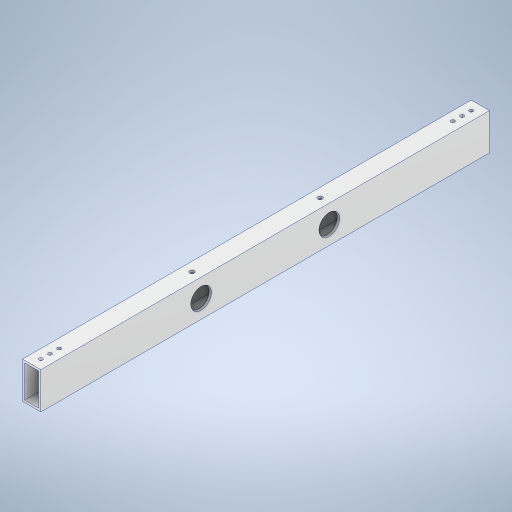
# Autodesk Inventor part: middle_alum_swerve
Saved by Autodesk Inventor 2024 (Build 280153000, 153)
## iProperties
Created: 2023-10-09
Part Number: middle_alum_swerve
Material: Aluminum 6061
Document SubType Name: Modeling
Designer: s137416
Density: 2.7 g/cm^3
Appearance: Aluminum - Flat
Author: s137416
Autodesk Inventor part; units mm, degrees
ref_plane "YZ Plane" through (0, 0, 0) normal (1, 0, 0) x (0, 1, 0)
ref_plane "XZ Plane" through (0, 0, 0) normal (0, 1, 0) x (-1, 0, 0)
ref_plane "XY Plane" through (0, 0, 0) normal (0, 0, 1) x (1, 0, 0)
sketch "Sketch1" plane through (0, 0, 0) normal (0, 1, 0) x (-1, 0, 0)
  line L0 (5.8164, 600.598) -> (-19.5836, 600.598)
  line L1 (-19.5836, 600.598) -> (-19.5836, -21.702)
  line L2 (-19.5836, -21.702) -> (5.8164, -21.702)
  line L3 (5.8164, -21.702) -> (5.8164, 600.598)
  point P0 (0, 0)
  dimension "d0" = 25.4
  dimension "d1" = 622.3
  constraints: 8 end point, 2 parallel, 1 horizontal, 1 perpendicular
  measures "d0" distance of L2.end L1.end
  measures "d1" distance of L2.end L0.start
extrude "Extrusion1" add sketch "Sketch1" along normal blind 50.8
shell "Shell1" thickness 3.175 removed faces 2 at (2.6503, 33.8667, 600.598) at (11.117, 33.8667, -21.702)
sketch "Sketch2" plane through (0, 50.8, 0) normal (0, 1, 0) x (1, 0, 0)
  circle A0 centre (6.8836, -587.898) radius 2.5019
  line L0 (-5.8164, -600.598) -> (19.5836, -600.598) projected
  circle A1 centre (6.8836, -575.198) radius 2.5019
  circle A2 centre (6.8836, -562.498) radius 2.5019
  circle A3 centre (6.8836, 9.002) radius 2.5019
  circle A4 centre (6.8836, -3.698) radius 2.5019
  circle A5 centre (6.8836, -16.398) radius 2.5019
  line L1 (19.5836, 21.702) -> (-5.8164, 21.702) projected
  point P0 (0, 0)
  dimension "d5" = 5.0038
  dimension "d6" = 12.7
  dimension "d7" = 5.0038
  dimension "d8" = 5.0038
  dimension "d9" = 12.7
  dimension "d10" = 12.7
  dimension "d11" = 5.0038
  dimension "d12" = 5.0038
  dimension "d13" = 5.0038
  dimension "d14" = 12.7
  dimension "d15" = 12.7
  dimension "d16" = 12.7
  constraints: 6 centre point
  measures "d5" diameter of A0
  measures "d6" distance from line of L0 A0.centre
  measures "d7" diameter of A1
  measures "d8" diameter of A2
  measures "d9" distance of A0.centre A1.centre
  measures "d10" distance of A1.centre A2.centre
  measures "d11" diameter of A3
  measures "d12" diameter of A4
  measures "d13" diameter of A5
  measures "d14" distance from line of L1 A3.centre
  measures "d15" distance of A4.centre A3.centre
  measures "d16" distance of A4.centre A5.centre
extrude "Extrusion2" cut sketch "Sketch2" against normal blind 50.8
sketch "Sketch3" plane through (19.5836, 0, 600.598) normal (1, 0, 0) x (0, 0, -1)
  line L0 (0, 0) -> (0, 50.8) construction
  line L1 (622.3, 0) -> (622.3, 50.8) construction
  circle A0 centre (222.25, 25.4) radius 14.2875
  circle A1 centre (400.05, 25.4) radius 14.2875
  point P0 (600.598, 0)
  dimension "d21" = 28.575
  dimension "d22" = 28.575
  constraints: 2 centre point
  measures "d21" diameter of A0
  measures "d22" diameter of A1
hole "Hole1" at (19.5836, 25.4, 378.348) at (19.5836, 25.4, 200.548) direction (-1, 0, 0) diameter 28.575 end through all
sketch "Sketch4" plane through (0, 50.8, 0) normal (0, 1, 0) x (1, 0, 0)
  circle A0 centre (6.8836, -378.348) radius 3.175
  line L0 (-5.8164, -600.598) -> (19.5836, -600.598) projected
  circle A1 centre (6.8836, -200.548) radius 3.175
  line L1 (19.5836, 21.702) -> (-5.8164, 21.702) projected
  point P0 (0, 0)
  point P1 (6.8836, -600.598)
  dimension "d30" = 6.35
  dimension "d31" = 222.25
  dimension "d32" = 6.35
  dimension "d33" = 222.25
  constraints: 2 centre point, 1 midpoint
  measures "d30" diameter of A0
  measures "d31" distance of point (6.884, -600.598) A0.centre
  measures "d32" diameter of A1
  measures "d33" distance from line of L1 A1.centre
hole "Hole2" at (6.8836, 50.8, 378.348) at (6.8836, 50.8, 200.548) direction (0, -1, 0) diameter 6.35 end through all
body "Solid1"
